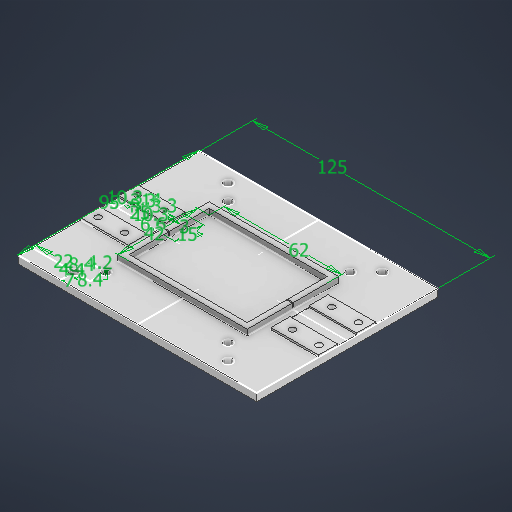
# Autodesk Inventor part: Molde grande 643FBR 1mm
Saved by Autodesk Inventor 2026.1 (Build 301233000, 233)
## iProperties
Created: 2025-11-18
Part Number: Molde grande 643FBR 1mm
Material: Genérico
Document SubType Name: Modeling
Designer: Laboratorio_sensores
Density: 1 g/cm^3
Appearance: Valor por defecto
Author: Laboratorio_sensores
Autodesk Inventor part; units mm, degrees
ref_plane "YZ Plane" through (0, 0, 0) normal (1, 0, 0) x (0, 1, 0)
ref_plane "XZ Plane" through (0, 0, 0) normal (0, 1, 0) x (-1, 0, 0)
ref_plane "XY Plane" through (0, 0, 0) normal (0, 0, 1) x (1, 0, 0)
sketch "Boceto1" plane through (0, 0, 0) normal (0, 1, 0) x (-1, 0, 0)
  line L0 (0, 0) -> (125, 0)
  line L1 (125, 0) -> (125, -95)
  line L2 (125, -95) -> (0, -95)
  line L3 (0, -95) -> (0, 0)
  line L4 (93.5, -26.5) -> (31.5, -26.5)
  line L5 (31.5, -26.5) -> (31.5, -68.5)
  line L6 (31.5, -68.5) -> (93.5, -68.5)
  line L7 (93.5, -68.5) -> (93.5, -26.5)
  line L8 (62.5, -26.5) -> (62.5, 0)
  line L9 (93.5, -47.5) -> (125, -47.5)
  line L10 (62.5, -68.5) -> (62.5, -95)
  line L11 (31.5, -47.5) -> (0, -47.5)
  line L12 (96.5, -23.5) -> (28.5, -23.5)
  line L13 (28.5, -23.5) -> (28.5, -71.5)
  line L14 (28.5, -71.5) -> (96.5, -71.5)
  line L15 (96.5, -71.5) -> (96.5, -23.5)
  line L16 (125, 0) -> (103, 0)
  line L17 (103, 0) -> (103, -7)
  line L18 (103, -7) -> (125, -7)
  line L19 (125, -7) -> (125, 0)
  circle A0 centre (103, -7) radius 2.2
  circle A1 centre (103, -88) radius 2.2
  circle A2 centre (22, -7) radius 2.2
  circle A3 centre (22, -88) radius 2.2
  line L20 (125, -47.5) -> (100, -47.5)
  line L21 (100, -47.5) -> (100, -62.5)
  line L22 (100, -62.5) -> (125, -62.5)
  line L23 (100, -47.5) -> (100, -32.5)
  line L24 (100, -32.5) -> (125, -32.5)
  line L25 (120.6, -47.5) -> (120.6, -57.8)
  circle A4 centre (120.6, -57.8) radius 1.65
  circle A5 centre (120.6, -37.2) radius 1.65
  line L26 (25, -47.5) -> (25, -62.5)
  line L27 (25, -62.5) -> (0, -62.5)
  line L28 (25, -47.5) -> (25, -32.5)
  line L29 (25, -32.5) -> (0, -32.5)
  circle A6 centre (4.4, -57.8) radius 1.65
  circle A7 centre (4.4, -37.2) radius 1.65
  line L30 (103, -7) -> (94.6, -7)
  line L31 (103, -7) -> (103, -15.4)
  line L32 (103, -7) -> (94.6, -7)
  line L33 (94.6, -7) -> (94.6, -15.4)
  line L34 (94.6, -15.4) -> (103, -15.4)
  line L35 (103, -15.4) -> (103, -7)
  circle A8 centre (94.6, -15.4) radius 2.1
  circle A9 centre (94.6, -79.6) radius 2.1
  circle A10 centre (30.4, -15.4) radius 2.1
  circle A11 centre (30.4, -79.6) radius 2.1
  line L36 (106.6, -47.5) -> (106.6, -57.8)
  circle A12 centre (106.6, -57.8) radius 1.65
  circle A13 centre (106.6, -37.2) radius 1.65
  circle A14 centre (18.4, -57.8) radius 1.65
  circle A15 centre (18.4, -37.2) radius 1.65
  point P0 (62.5, -23.5)
  point P1 (62.5, -71.5)
  dimension "d0" = 95
  dimension "d1" = 125
  dimension "d2" = 42
  dimension "d3" = 62
  dimension "d4" = 3
  dimension "d5" = 7
  dimension "d6" = 22
  dimension "d7" = 4.4
  dimension "d10" = 25
  dimension "d11" = 15
  dimension "d12" = 10.3
  dimension "d13" = 3.3
  dimension "d29" = 8.4
  dimension "d30" = 8.4
  dimension "d31" = 4.2
  dimension "d35" = 10.3
  dimension "d36" = 3.3
  dimension "d37" = 6.6
  dimension "d38" = 14
  constraints: 74 end point, 18 symmetric about line, 16 centre point, 12 perpendicular, 11 parallel, 8 midpoint, 4 coincident, 4 horizontal, 4 point on line, 3 vertical, 15 other
  measures "d0" distance of L0.end L1.end
  measures "d1" distance of L1.end L2.end
  measures "d2" distance of L6.end L4.start
  measures "d3" distance of L5.end L6.end
  measures "d4" distance between parallel lines of L15 L7
  measures "d5" distance of L16.end L17.end
  measures "d6" distance of L17.end L18.end
  measures "d7" diameter of A0
  measures "d10" distance of L9.end L20.end
  measures "d11" distance of L20.end L21.end
  measures "d12" distance of L25.start L25.end
  measures "d13" diameter of A4
  measures "d29" distance of L30.start L30.end
  measures "d30" distance of L30.start L31.end
  measures "d31" diameter of A8
  measures "d35" distance of L36.start L36.end
  measures "d36" diameter of A12
  measures "d37" distance between parallel lines of L36 L21
  measures "d38" distance of L25.end L36.end
extrude "Extrusión1" add sketch "Boceto1" against normal blind 4 contours L0 L8 L12 L13 L11 L28 L29 L3 | L0 L17 A0 L30 L33 A8 L34 L31 L18 L1 L24 L23 L9 L15 L12 L8 | L29 L28 L11 L3 | L0 L1 L18 A0 L17 | L12 L15 L9 L7 L4 L8 | L8 L4 L5 L11 L13 L12 | L11 L26 L27 L3 | L4 L7 L6 L5 | L27 L26 L11 L13 L14 L10 L2 L3 | A0 L31 L34 A8 L33 L30 | L15 L14 L10 L6 L7 L9 | L9 L21 L22 L1 L2 L10 L14 L15 | L11 L5 L6 L10 L14 L13 | L1 L9 L23 L24 | A12 | L9 L1 L22 L21 | A8 L34 L33 | L33 L34 A8 | A9 | A10 | A11 | A13 | A14 | A15
extrude "Extrusión2" add sketch "Boceto1" along normal blind 3 contours L12 L15 L9 L7 L4 L8 | L8 L4 L5 L11 L13 L12 | L15 L14 L10 L6 L7 L9 | L11 L5 L6 L10 L14 L13
sketch "Boceto2" plane through (0, 3, 0) normal (0, 1, 0) x (1, 0, 0)
  line L0 (-31.5, 47.5) -> (0, 47.5) projected
  line L1 (-62.5, 68.5) -> (-62.5, 95) projected
  line L2 (-28.5, 23.5) -> (-28.5, 71.5) projected
  line L3 (-31.5, 68.5) -> (-31.5, 26.5) projected
  line L4 (-28.5, 47.25) -> (-31.5, 47.25)
  line L5 (-31.5, 47.25) -> (-31.5, 47.75)
  line L6 (-31.5, 47.75) -> (-28.5, 47.75)
  line L7 (-28.5, 47.75) -> (-28.5, 47.25)
  line L8 (-96.5, 23.5) -> (-96.5, 71.5)
  line L9 (-93.5, 68.5) -> (-93.5, 26.5)
  line L10 (-96.5, 47.25) -> (-93.5, 47.25)
  line L11 (-93.5, 47.75) -> (-96.5, 47.75)
  point P0 (0, 0)
  point P1 (-93.5, 47.25)
  point P2 (-96.5, 47.75)
  point P3 (-31.5, 47.25)
  point P4 (-28.5, 47.75)
  dimension "d16" = 0.5
  dimension "d17" = 0.25
  constraints: 16 end point, 8 symmetric about line, 4 point on line, 2 parallel, 1 horizontal, 1 perpendicular
  measures "d16" distance between parallel lines of L4 L6
  measures "d17" distance between parallel lines of L0 L6
extrude "Extrusión3" cut sketch "Boceto2" against normal blind 2
extrude "Extrusión4" add sketch "Boceto1" along normal blind 1 contours L29 L28 L11 L3 | L11 L26 L27 L3 | L1 L9 L23 L24 | A12 | L9 L1 L22 L21 | A13 | A14 | A15
sketch "Boceto3" plane through (0, 1, 0) normal (0, 1, 0) x (1, 0, 0)
  line L0 (-31.5, 47.5) -> (0, 47.5) projected
  line L1 (-25, 62.5) -> (-25, 32.5) projected
  line L2 (0, 32.5) -> (0, 62.5) projected
  line L3 (-25, 42.5) -> (0, 42.5)
  line L4 (0, 42.5) -> (0, 52.5)
  line L5 (0, 52.5) -> (-25, 52.5)
  line L6 (-25, 52.5) -> (-25, 42.5)
  line L7 (-62.5, 68.5) -> (-62.5, 95) projected
  line L8 (-100, 62.5) -> (-100, 32.5)
  line L9 (-125, 32.5) -> (-125, 62.5)
  line L10 (-100, 42.5) -> (-125, 42.5)
  line L11 (-125, 52.5) -> (-100, 52.5)
  point P0 (0, 0)
  point P1 (-125, 42.5)
  point P2 (-100, 52.5)
  point P3 (0, 42.5)
  point P4 (-25, 52.5)
  dimension "d22" = 5
  dimension "d23" = 5
  constraints: 16 end point, 8 symmetric about line, 4 point on line, 2 parallel, 1 horizontal, 1 perpendicular
  measures "d22" distance between parallel lines of L3 L0
  measures "d23" distance between parallel lines of L5 L0
extrude "Extrusión5" cut sketch "Boceto3" against normal blind 0.8
sketch "Boceto4" plane through (0, -4, 0) normal (0, -1, 0) x (1, 0, 0)
  circle A0 centre (-4.4, -37.2) radius 1.65 projected
  line L0 (-1.2823, -37.2) -> (-2.8412, -39.9)
  line L1 (-2.8412, -39.9) -> (-5.9588, -39.9)
  line L2 (-5.9588, -39.9) -> (-7.5177, -37.2)
  line L3 (-7.5177, -37.2) -> (-5.9588, -34.5)
  line L4 (-5.9588, -34.5) -> (-2.8412, -34.5)
  line L5 (-2.8412, -34.5) -> (-1.2823, -37.2)
  line L6 (-31.5, -47.5) -> (0, -47.5) projected
  line L7 (-62.5, -68.5) -> (-62.5, -95) projected
  line L8 (-1.2823, -57.8) -> (-2.8412, -55.1)
  line L9 (-2.8412, -55.1) -> (-5.9588, -55.1)
  line L10 (-5.9588, -55.1) -> (-7.5177, -57.8)
  line L11 (-7.5177, -57.8) -> (-5.9588, -60.5)
  line L12 (-5.9588, -60.5) -> (-2.8412, -60.5)
  line L13 (-2.8412, -60.5) -> (-1.2823, -57.8)
  line L14 (-123.7177, -37.2) -> (-122.1588, -39.9)
  line L15 (-122.1588, -39.9) -> (-119.0412, -39.9)
  line L16 (-119.0412, -39.9) -> (-117.4823, -37.2)
  line L17 (-117.4823, -37.2) -> (-119.0412, -34.5)
  line L18 (-119.0412, -34.5) -> (-122.1588, -34.5)
  line L19 (-122.1588, -34.5) -> (-123.7177, -37.2)
  line L20 (-122.1588, -60.5) -> (-123.7177, -57.8)
  line L21 (-123.7177, -57.8) -> (-122.1588, -55.1)
  line L22 (-122.1588, -55.1) -> (-119.0412, -55.1)
  line L23 (-119.0412, -55.1) -> (-117.4823, -57.8)
  line L24 (-117.4823, -57.8) -> (-119.0412, -60.5)
  line L25 (-119.0412, -60.5) -> (-122.1588, -60.5)
  line L26 (-4.4, -57.8) -> (-18.4, -57.8)
  line L27 (-18.4, -57.8) -> (-11.4, -57.8)
  line L28 (-11.4, -60.5) -> (-11.4, -57.8)
  line L29 (-4.4, -37.2) -> (-18.4, -37.2)
  line L30 (-18.4, -37.2) -> (-11.4, -37.2)
  line L31 (-11.4, -37.2) -> (-11.4, -39.9)
  line L32 (-21.5177, -37.2) -> (-19.9588, -39.9)
  line L33 (-19.9588, -39.9) -> (-16.8412, -39.9)
  line L34 (-16.8412, -39.9) -> (-15.2823, -37.2)
  line L35 (-15.2823, -37.2) -> (-16.8412, -34.5)
  line L36 (-16.8412, -34.5) -> (-19.9588, -34.5)
  line L37 (-19.9588, -34.5) -> (-21.5177, -37.2)
  line L38 (-19.9588, -60.5) -> (-21.5177, -57.8)
  line L39 (-21.5177, -57.8) -> (-19.9588, -55.1)
  line L40 (-19.9588, -55.1) -> (-16.8412, -55.1)
  line L41 (-16.8412, -55.1) -> (-15.2823, -57.8)
  line L42 (-15.2823, -57.8) -> (-16.8412, -60.5)
  line L43 (-16.8412, -60.5) -> (-19.9588, -60.5)
  line L44 (-108.1588, -60.5) -> (-105.0412, -60.5)
  line L45 (-105.0412, -60.5) -> (-103.4823, -57.8)
  line L46 (-103.4823, -57.8) -> (-105.0412, -55.1)
  line L47 (-105.0412, -55.1) -> (-108.1588, -55.1)
  line L48 (-108.1588, -55.1) -> (-109.7177, -57.8)
  line L49 (-109.7177, -57.8) -> (-108.1588, -60.5)
  line L50 (-109.7177, -37.2) -> (-108.1588, -34.5)
  line L51 (-108.1588, -39.9) -> (-109.7177, -37.2)
  line L52 (-105.0412, -39.9) -> (-108.1588, -39.9)
  line L53 (-103.4823, -37.2) -> (-105.0412, -39.9)
  line L54 (-105.0412, -34.5) -> (-103.4823, -37.2)
  line L55 (-108.1588, -34.5) -> (-105.0412, -34.5)
  point P0 (0, 0)
  point P1 (-4.4, -39.9)
  point P2 (-4.4, -34.5)
  point P3 (-120.6, -39.9)
  point P4 (-106.6, -57.8)
  point P5 (-106.6, -37.2)
  dimension "d26" = 5.4
  constraints: 108 end point, 43 symmetric about line, 4 midpoint, 2 horizontal, 1 coincident, 1 perpendicular, 1 point on line, 13 other
  measures "d26" distance of point (-4.4, -39.9) point (-4.4, -34.5)
extrude "Extrusión6" cut sketch "Boceto4" against normal blind 2.5 contours A0 | L3 L4 L5 L0 L1 L2 | L34 L33 L32 L37 L36 L35 | L13 L12 L11 L10 L9 L8 | L42 L43 L38 L39 L40 L41 | L19 L18 L17 L16 L15 L14 | L20 L21 L22 L23 L24 L25 | L49 L48 L47 L46 L45 L44 | L50 L55 L54 L53 L52 L51
extrude "Extrusión7" cut sketch "Boceto1" against normal blind 5 contours A8 L34 L33 | L33 L34 A8 | A9 | A10 | A11
extrude "Extrusión8" cut sketch "Boceto1" along normal mid plane 10 contours A12 | A13 | A14 | A15
equation "\"d36\" = d13"
